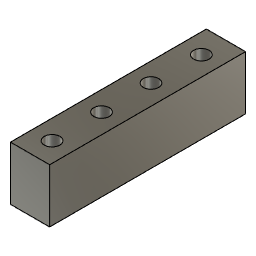
LedTaster_4TE_Positionierer (Autodesk Fusion 360 design; units mm, degrees)
Autodesk Fusion 360 part; units mm, degrees
note: some values were not read from the file. Set by a fixed rule: which sketch regions a step uses.
sketch "Sketch1" plane through (0, 0, 0) normal (0, 0, 1) x (1, 0, 0)
  line L0 (0, 0) -> (8, 0)
  line L1 (8, 0) -> (8, 40)
  line L2 (8, 40) -> (0, 40)
  line L3 (0, 40) -> (0, 0)
  circle A0 centre (4, 4.495) radius 1.575
  circle A1 centre (4, 4.495) radius 1.875
  circle A2 centre (3.9787, 14.6137) radius 1.575
  circle A3 centre (3.8912, 24.7987) radius 1.575
  circle A4 centre (4.0306, 34.9431) radius 1.575
  circle A5 centre (3.9787, 14.6137) radius 1.875
  circle A6 centre (3.8912, 24.7987) radius 1.875
  circle A7 centre (4.0306, 34.9431) radius 1.875
  point P0 (3.8912, 24.7987)
  point P1 (4.0306, 34.9431)
  point P2 (3.9787, 14.6137)
  point P3 (4, 4.495)
  dimension "d1" = 3.15
  dimension "d2" = 0.3
  dimension "d11" = 40
  dimension "d12" = 4
  dimension "d13" = 8
  dimension "d14" = 4.495
  dimension "d15" = 14.6137
  dimension "d16" = 24.7987
  dimension "d17" = 34.9431
  constraint coincident P3 A0.centre
  constraint coincident P2 A2.centre
  constraint coincident P0 A3.centre
  constraint coincident P1 A4.centre
  constraint equal A0 A2
  constraint equal A2 A3
  constraint equal A3 A4
  constraint equal A1 A5
  constraint equal A5 A6
  constraint equal A6 A7
  measures "d1" diameter of A0
  measures "d11" distance of L0.start L2.end
  measures "d12" horizontal distance of L0.start P3
  measures "d13" distance of L0.start L0.end
  measures "d14" vertical distance of L0.start P3
  measures "d15" vertical distance of L0.start P2
  measures "d16" vertical distance of L0.start A3.centre
  measures "d17" vertical distance of L0.start P1
extrude "Extrude1" add sketch "Sketch1" against normal blind 3.6 contours L0 L1 L2 L3 | A1 | A5 | A6 | A7
fillet "Fillet1" radius 0.5 4 edges at (2.5316, 3.9255, -3.6) (2.5103, 14.0442, -3.6) (2.4228, 24.2292, -3.6) (2.5622, 34.3736, -3.6)
extrude "Extrude2" add sketch "Sketch1" against normal blind 11 contours L0 L1 L2 L3
fillet "Fillet2" radius 1 4 edges at (2.2519, 3.817, -11) (2.2306, 13.9357, -11) (2.1431, 24.1207, -11) (2.2825, 34.2651, -11)
equation "d13 = d12 * 2"
